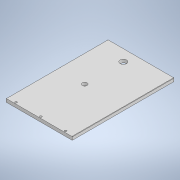
# Autodesk Inventor part: płyta_boczna_obudowy
Saved by Autodesk Inventor 2020 (Build 240168000, 168)
## iProperties
Created: 2020-08-21
Part Number: płyta_boczna_obudowy
Material: Generic
Document SubType Name: Modeling
Designer: Hesekiel
Density: 1 g/cm^3
Appearance: Default
Author: Hesekiel
Autodesk Inventor part; units mm, degrees
ref_plane "YZ Plane" through (0, 0, 0) normal (1, 0, 0) x (0, 1, 0)
ref_plane "XZ Plane" through (0, 0, 0) normal (0, 1, 0) x (-1, 0, 0)
ref_plane "XY Plane" through (0, 0, 0) normal (0, 0, 1) x (1, 0, 0)
sketch "Sketch1" plane through (0, 0, 0) normal (0, 1, 0) x (-1, 0, 0)
  line L0 (102.5, 157.5) -> (-102.5, 157.5)
  line L1 (-102.5, 157.5) -> (-102.5, -157.5)
  line L2 (-102.5, -157.5) -> (102.5, -157.5)
  line L3 (102.5, -157.5) -> (102.5, 157.5)
  line L4 (102.5, 157.5) -> (-102.5, -157.5) construction
  line L5 (-102.5, 157.5) -> (102.5, -157.5) construction
  point P0 (0, 0)
  dimension "d0" = 205
  dimension "d1" = 315
  constraints: 12 end point, 2 midpoint, 2 parallel, 1 horizontal, 1 perpendicular
  measures "d0" distance of L2.end L1.end
  measures "d1" distance of L1.end L0.end
extrude "Extrusion1" add sketch "Sketch1" along normal blind 10
fillet "Fillet1" radius 1 2 edges at (102.5, 10, 0) (-102.5, 10, 0)
sketch "Sketch3" plane through (0, 0, 0) normal (0, -1, 0) x (1, 0, 0)
  line L0 (102.5, -157.5) -> (-102.5, -157.5) projected
  line L1 (102.5, 157.5) -> (102.5, -157.5) projected
  line L2 (-102.5, 157.5) -> (102.5, 157.5) projected
  line L3 (-102.5, -157.5) -> (-102.5, 157.5) projected
  line L4 (102.5, 157.5) -> (102.5, -157.5) projected
  line L5 (-102.5, -157.5) -> (-102.5, 157.5) projected
  line L6 (102.5, 157.5) -> (-102.5, 157.5)
  line L7 (-102.5, 157.5) -> (-102.5, 147.5)
  line L8 (-102.5, 147.5) -> (102.5, 147.5)
  line L9 (102.5, 147.5) -> (102.5, 157.5)
  line L10 (102.5, 152.5) -> (-102.5, 152.5)
  line L11 (102.5, 152.5) -> (0, 152.5)
  line L12 (51.25, 152.5) -> (102.5, 152.5)
  line L13 (0, 152.5) -> (-102.5, 152.5)
  line L14 (-102.5, 152.5) -> (-51.25, 152.5)
  circle A0 centre (76.875, 152.5) radius 3.3
  circle A1 centre (0, 152.5) radius 3.3
  circle A2 centre (-76.875, 152.5) radius 3.3
  point P0 (0, 0)
  dimension "d5" = 10
  dimension "d6" = 6.6
  dimension "d7" = 6.6
  dimension "d8" = 6.6
  constraints: 18 end point, 7 midpoint, 3 centre point, 2 horizontal, 2 parallel, 1 coincident, 1 collinear, 1 perpendicular, 1 point on line
  measures "d5" distance of L7.end L6.end
  measures "d6" diameter of A0
  measures "d7" diameter of A1
  measures "d8" diameter of A2
extrude "Extrusion2" cut sketch "Sketch3" against normal up to surface (10 mm away) contours A0 L10 | L10 A0 | A2 L10 | L10 A2 | A1 L10 | L10 A1
sketch "Sketch4" plane through (0, 10, 0) normal (0, 1, 0) x (1, 0, 0)
  line L0 (-101.5, -157.5) -> (-102.5, -157.5) projected
  line L1 (-102.5, -157.5) -> (-19, -157.5)
  line L2 (-101.5, -157.5) -> (101.5, -157.5) projected
  line L3 (-19, -157.5) -> (-19, 2.5)
  circle A0 centre (-19, 2.5) radius 7.5
  line L4 (-19, 2.5) -> (-19, 122.5)
  circle A1 centre (-19, 122.5) radius 10
  point P0 (0, 0)
  dimension "d11" = 83.5
  dimension "d12" = 160
  dimension "d13" = 15
  dimension "d16" = 120
  dimension "d17" = 20
  constraints: 6 end point, 2 centre point, 2 coincident, 1 perpendicular, 1 point on line, 1 vertical
  measures "d11" distance of L0.end L1.end
  measures "d12" distance of L1.end L3.end
  measures "d13" diameter of A0
  measures "d16" distance of L4.start L4.end
  measures "d17" diameter of A1
extrude "Extrusion3" cut sketch "Sketch4" against normal up to surface (10 mm away) contours A0 L4 L3 | L3 L4 A0
extrude "Extrusion4" cut sketch "Sketch4" against normal up to surface (10 mm away) contours A1
body "Solid1"
